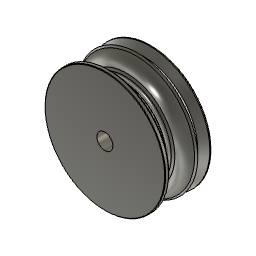
Wheel v3 (Autodesk Fusion 360 design; units mm, degrees)
Autodesk Fusion 360 part; units mm, degrees
sketch "Sketch1" plane through (0, 0, 0) normal (1, 0, 0) x (0, 1, 0)
  line L0 (0, 0) -> (9.2, 0)
  line L1 (9.2, 0) -> (9.2, 12)
  line L2 (9.2, 12) -> (0, 12)
  line L3 (0, 12) -> (0, 0)
  line L4 (0, 10.3) -> (9.2, 10.3)
  line L5 (7.1, 0) -> (8.3, 0)
  line L6 (8.3, 0) -> (8.3, 1.2)
  line L7 (8.3, 1.2) -> (7.1, 1.2)
  line L8 (7.1, 1.2) -> (7.1, 0)
  circle A0 centre (3.6, 0) radius 2.6
  line L9 (3.6, 0) -> (3.6, 2.6) construction
  circle A1 centre (3.6, 2.6) radius 0.5
  dimension "d1" = 9.2
  dimension "d2" = 12
  dimension "d3" = 1.7
  dimension "d4" = 1.2
  dimension "d5" = 1.2
  dimension "d6" = 7.1
  dimension "d7" = 5.2
  dimension "d8" = 3.6
  dimension "d9" = 1
  constraint horizontal L0
  constraint vertical L1
  constraint horizontal L2
  constraint vertical L3
  constraint coincident L0.start L3.end
  constraint coincident L3 L4.start
  constraint coincident L1 L4.end
  constraint perpendicular L1 L4
  constraint horizontal L5
  constraint vertical L6
  constraint horizontal L7
  constraint vertical L8
  constraint coincident L0 L5.start
  constraint coincident L0 A0.centre
  constraint coincident A0.centre L9.start
  constraint coincident A0 L9.end
  constraint perpendicular L0 L9
  constraint coincident L9.end A1.centre
  measures "d1" distance of L0.start L0.end
  measures "d2" distance of L0.start L2.end
  measures "d3" distance of L2 L4
  measures "d4" distance of L5.start L5.end
  measures "d5" distance of L5.start L7.end
  measures "d6" distance of L3 L8
  measures "d7" diameter of A0
  measures "d8" distance of L3 A0.centre
  measures "d9" diameter of A1
revolve "Revolve1" add sketch "Sketch1" angle 360 about axis through (0, 9.2, 12) along (0, -1, 0) contours L0 L1 L3 L4 L6 L7 L8 A0 A1 | L1 L2 L3 L4
chamfer "Chamfer1" distance 0.6 angle 45 2 faces at (-0.5962, 7.1, 0.4447) (-1.1327, 8.3, 0.4849)
chamfer "Chamfer1" distance 0.1 angle 45 2 edges at (-11.1879, 9.2, 7.6606) (-11.1879, 0, 7.6606)
chamfer "Chamfer1" distance 0.28 distance2 0.31 2 edges at (-8.8087, 4.0977, 8.5834) (-8.8087, 3.1023, 8.5834) measured on face at (-3.6679, 4.0982, 20.7013) measured on face at (7.1736, 1.0027, 21.4704)
chamfer "Chamfer1" distance 0.32 distance2 0.3 2 edges at (-11.1879, 6.2, 7.6606) (-11.1879, 1, 7.6606) measured on face at (-1.1829, 6.1973, 23.8216) measured on face at (-0.5982, 0.3333, 0.0149)
sketch "Sketch2" plane through (0, 0, 0) normal (0, -1, 0) x (1, 0, 0)
  circle A0 centre (0, 12) radius 11.9
  circle A1 centre (0, 12) radius 1.6
  line L0 (0.0188, 10.4001) -> (0, 0) construction
  dimension "d17" = 3.2
  constraint concentric A0 A1
  constraint coincident A1 L0.start
  constraint coincident L0.end origin
  measures "d17" diameter of A1
extrude "Extrude1" cut sketch "Sketch2" against normal up to surface (9.2 mm away) contours A1
